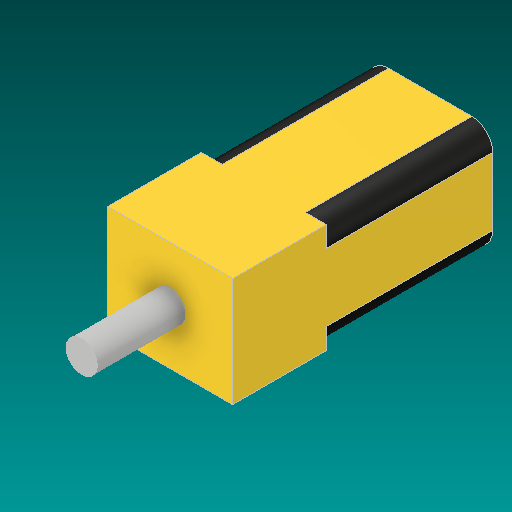
# Autodesk Inventor part: MicroMotor
Saved by Autodesk Inventor 2020 (Build 240168000, 168)
## iProperties
Created: 2019-12-04
Part Number: MicroMotor
Material: Generic
Document SubType Name: Modeling
Designer: Santiago
Density: 1 g/cm^3
Appearance: Default
Author: Santiago
Autodesk Inventor part; units mm, degrees
ref_plane "YZ Plane" through (0, 0, 0) normal (1, 0, 0) x (0, 1, 0)
ref_plane "XZ Plane" through (0, 0, 0) normal (0, 1, 0) x (-1, 0, 0)
ref_plane "XY Plane" through (0, 0, 0) normal (0, 0, 1) x (1, 0, 0)
sketch "Sketch1" plane through (0, 0, 0) normal (0, 0, 1) x (1, 0, 0)
  line L0 (0, 0) -> (12, 0)
  line L1 (12, 0) -> (12, 10.5)
  line L2 (12, 10.5) -> (0, 10.5)
  line L3 (0, 10.5) -> (0, 0)
  dimension "d0" = 12
  dimension "d2" = 10.5
  constraints: 8 end point, 2 perpendicular, 1 horizontal, 1 vertical
  measures "d0" distance of L0.start L0.end
  measures "d2" distance of L0.end L1.end
extrude "Extrusion1" add sketch "Sketch1" along normal blind 16
fillet "Fillet1" radius 2 4 edges at (12, 10.5, 8) (0, 10.5, 8) (12, 0, 8) (0, 0, 8)
sketch "Sketch2" plane through (0, 0, 16) normal (0, 0, 1) x (1, 0, 0)
  line L0 (12, 2) -> (12, 8.5) projected
  line L1 (10, 10.5) -> (2, 10.5) projected
  line L2 (0, 8.5) -> (0, 2) projected
  line L3 (2, 0) -> (10, 0) projected
  arc A0 (12, 8.5) -> (10, 10.5) centre (10, 8.5) ccw projected
  line L4 (12, 8.5) -> (12, 10.5)
  line L5 (12, 10.5) -> (10, 10.5)
  line L6 (2, 10.5) -> (0, 10.5)
  line L7 (0, 10.5) -> (0, 8.5)
  arc A1 (0, 2) -> (2, 0) centre (2, 2) ccw projected
  line L8 (2, 0) -> (0, 0)
  line L9 (0, 0) -> (2, 0)
  line L10 (12, 2) -> (12, 0)
  arc A2 (10, 0) -> (12, 2) centre (10, 2) ccw projected
  line L11 (12, 0) -> (10, 0)
  line L12 (0, 0) -> (0, 2)
  constraints: 18 end point, 5 tangent, 3 perpendicular, 2 collinear, 1 horizontal, 1 point on line, 1 vertical
extrude "Extrusion2" add sketch "Sketch2" along normal blind 9
sketch "Sketch3" plane through (0, 0, 25) normal (0, 0, 1) x (1, 0, 0)
  line L0 (10, 10.5) -> (2, 10.5) projected
  line L1 (6, 10.5) -> (6, 0)
  line L2 (2, 0) -> (10, 0) projected
  circle A0 centre (6, 5.25) radius 1.5
  point P0 (0, 0)
  dimension "d8" = 3
  constraints: 3 midpoint, 2 end point, 1 centre point
  measures "d8" diameter of A0
extrude "Extrusion3" add sketch "Sketch3" along normal blind 8.5
body "Solid1"
